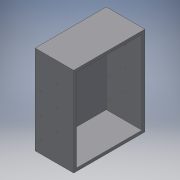
# Autodesk Inventor part: Cart Box
Saved by Autodesk Inventor 2018 (Build 220112000, 112)
## iProperties
Created: 2018-12-10
Part Number: Cart Box
Material: Generic
Document SubType Name: Modeling
Designer: Gabriel
Density: 1 g/cm^3
Appearance: Default
Author: Gabriel
Autodesk Inventor part; units mm, degrees
ref_plane "YZ Plane" through (0, 0, 0) normal (1, 0, 0) x (0, 1, 0)
ref_plane "XZ Plane" through (0, 0, 0) normal (0, 1, 0) x (-1, 0, 0)
ref_plane "XY Plane" through (0, 0, 0) normal (0, 0, 1) x (1, 0, 0)
sketch "Sketch1" plane through (0, 0, 0) normal (1, 0, 0) x (0, 1, 0)
  line L0 (6.7738, 9.1186) -> (-882.2262, 9.1186)
  line L1 (-882.2262, 9.1186) -> (-882.2262, -600.4814)
  line L2 (-882.2262, -600.4814) -> (6.7738, -600.4814)
  line L3 (6.7738, -600.4814) -> (6.7738, 9.1186)
  line L4 (-18.6262, -16.2814) -> (-856.8262, -16.2814)
  line L5 (-856.8262, -16.2814) -> (-856.8262, -575.0814)
  line L6 (-856.8262, -575.0814) -> (-18.6262, -575.0814)
  line L7 (-18.6262, -575.0814) -> (-18.6262, -16.2814)
  point P0 (0, 0)
  dimension "d0" = 889
  dimension "d1" = 609.6
  dimension "d2" = 25.4
  constraints: 16 end point, 4 parallel, 2 perpendicular, 1 horizontal, 3 other
  measures "d0" distance of L2.end L1.end
  measures "d1" distance of L1.end L0.end
  measures "d2" distance between parallel lines of L3 L7
extrude "Extrusion3" add sketch "Sketch1" along normal blind 304.8
sketch "Sketch4" plane through (0, 0, 0) normal (-1, 0, 0) x (0, 0, 1)
  line L0 (9.1186, 6.7738) -> (9.1186, -882.2262) projected
  line L1 (9.1186, -882.2262) -> (-600.4814, -882.2262) projected
  line L2 (9.1186, 6.7738) -> (-600.4814, 6.7738)
  line L3 (-600.4814, 6.7738) -> (-600.4814, -882.2262)
  line L4 (-600.4814, -882.2262) -> (9.1186, -882.2262)
  line L5 (9.1186, -882.2262) -> (9.1186, 6.7738)
  point P0 (0, 0)
  constraints: 8 end point, 2 parallel, 1 horizontal, 1 perpendicular
extrude "Extrusion4" add sketch "Sketch4" along normal blind 25.4
sketch "Sketch5" plane through (304.8, -882.2262, -600.4814) normal (0, 0, -1) x (-1, 0, 0)
  line L0 (0, 889) -> (330.2, 889) projected
  line L1 (330.2, 889) -> (330.2, 645.5901)
  line L2 (330.2, 889) -> (330.2, 0) projected
  line L3 (330.2, 457.2) -> (330.2, 279.4)
  line L4 (330.2, 279.4) -> (330.2, 101.6)
  line L5 (330.2, 518.5901) -> (609.6, 518.5901) construction
  line L6 (330.2, 340.7901) -> (609.6, 340.7901) construction
  line L7 (330.2, 162.9901) -> (609.6, 162.9901) construction
  line L8 (330.2, 457.2) -> (280.1718, 466.0213)
  line L9 (330.2, 457.2) -> (381, 457.2) construction
  line L10 (330.2, 279.4) -> (280.1718, 288.2213)
  line L11 (330.2, 279.4) -> (381, 279.4) construction
  line L12 (330.2, 101.6) -> (280.1718, 110.4213)
  line L13 (330.2, 101.6) -> (381, 101.6) construction
  line L14 (330.2, 0) -> (0, 0) projected
  line L15 (330.2, 0) -> (330.2, 101.6)
  circle A0 centre (280.1718, 466.0213) radius 2.5797
  circle A1 centre (280.1718, 288.2213) radius 2.5797
  circle A2 centre (280.1718, 110.4213) radius 2.5797
  line L16 (330.2, 457.2) -> (142.9418, 588.3196)
  line L17 (330.2, 457.2) -> (558.8, 457.2) construction
  line L18 (330.2, 279.4) -> (142.9418, 410.5196)
  line L19 (330.2, 279.4) -> (558.8, 279.4) construction
  line L20 (330.2, 101.6) -> (142.9418, 232.7196)
  line L21 (330.2, 101.6) -> (558.8, 101.6) construction
  circle A3 centre (142.9418, 588.3196) radius 2.5797
  circle A4 centre (142.9418, 410.5196) radius 2.5797
  circle A5 centre (142.9418, 232.7196) radius 2.5797
  point P0 (304.8, 882.2262)
  dimension "d16" = 177.8
  dimension "d17" = 177.8
  dimension "d35" = 50.8
  dimension "d36" = 170
  dimension "d37" = 50.8
  dimension "d38" = 170
  dimension "d39" = 50.8
  dimension "d40" = 170
  dimension "d46" = 101.6
  dimension "d48" = 5.1594
  dimension "d50" = 5.1594
  dimension "d52" = 5.1594
  dimension "d53" = 228.6
  dimension "d54" = 145
  dimension "d55" = 228.6
  dimension "d56" = 145
  dimension "d57" = 228.6
  dimension "d58" = 145
  dimension "d59" = 5.1594
  dimension "d60" = 5.1594
  dimension "d61" = 5.1594
  constraints: 38 end point, 9 horizontal, 6 centre point, 6 coincident, 6 equal length, 3 parallel, 1 point on line
  measures "d16" distance of L3.start L3.end
  measures "d17" distance of L3.end L4.end
  measures "d35" distance of L3.start L8.end
  measures "d36" angle of L9 L8
  measures "d37" distance of L3.end L10.end
  measures "d38" angle of L11 L10
  measures "d39" distance of L4.end L12.end
  measures "d40" angle of L13 L12
  measures "d46" distance of L2.end L15.end
  measures "d48" diameter of A0
  measures "d50" diameter of A1
  measures "d52" diameter of A2
  measures "d53" distance of L3.start L16.end
  measures "d54" angle of L17 L16
  measures "d55" distance of L3.end L18.end
  measures "d56" angle of L19 L18
  measures "d57" distance of L15.end L20.end
  measures "d58" angle of L21 L20
  measures "d59" diameter of A3
  measures "d60" diameter of A4
  measures "d61" diameter of A5
extrude "Extrusion6" cut sketch "Sketch5" against normal blind 914.4
body "Solid1"
